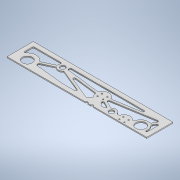
# Autodesk Inventor part: Right left side
Saved by Autodesk Inventor 2021 (Build 250183000, 183)
## iProperties
Created: 2020-09-02
Part Number: Right left side
Material: Generic
Document SubType Name: Modeling
Designer: deli
Density: 1 g/cm^3
Appearance: Default
Author: deli
Autodesk Inventor part; units mm, degrees
ref_plane "YZ Plane" through (0, 0, 0) normal (1, 0, 0) x (0, 1, 0)
ref_plane "XZ Plane" through (0, 0, 0) normal (0, 1, 0) x (-1, 0, 0)
ref_plane "XY Plane" through (0, 0, 0) normal (0, 0, 1) x (1, 0, 0)
sketch "Sketch1" plane through (0, 0, 0) normal (0, 1, 0) x (-1, 0, 0)
  arc A0 (82.9131, -43.5291) -> (113.1279, -37.6957) centre (96.2781, -31.587) ccw
  arc A1 (116.2464, -35.6057) -> (113.1279, -37.6957) centre (116.1128, -38.7779) ccw
  line L0 (116.2464, -35.6057) -> (118.6042, -35.705)
  arc A2 (121.4505, -37.7814) -> (118.6042, -35.705) centre (118.4706, -38.8772) ccw
  arc A3 (121.4505, -37.7814) -> (142.7671, -43.2201) centre (133.978, -33.1745) ccw
  arc A4 (146.2603, -42.7612) -> (142.7671, -43.2201) centre (144.8577, -45.6096) ccw
  line L1 (146.2603, -42.7612) -> (165.8088, -52.3866)
  arc A5 (167.5414, -55.7362) -> (165.8088, -52.3866) centre (164.4062, -55.235) ccw
  arc A6 (167.5414, -55.7362) -> (167.4812, -56.1422) centre (185.6904, -58.637) ccw
  arc A7 (164.8504, -58.8442) -> (167.4812, -56.1422) centre (164.3356, -55.7112) ccw
  line L2 (164.8504, -58.8442) -> (44.4643, -78.6278)
  arc A8 (41.2217, -73.8701) -> (44.4643, -78.6278) centre (43.9495, -75.4948) ccw
  line L3 (41.2217, -73.8701) -> (47.7775, -62.8629)
  arc A9 (51.3513, -61.4274) -> (47.7775, -62.8629) centre (50.5053, -64.4876) ccw
  arc A10 (51.3513, -61.4274) -> (77.4222, -45.0742) centre (56.9081, -41.3279) ccw
  arc A11 (82.9131, -43.5291) -> (77.4222, -45.0742) centre (80.5456, -45.6446) ccw
  line L4 (301.7886, -83.9745) -> (89.9873, -83.9745)
  arc A12 (89.4725, -77.6666) -> (89.9873, -83.9745) centre (89.9873, -80.7995) ccw
  line L5 (89.4725, -77.6666) -> (165.8801, -65.1101)
  arc A13 (169.2372, -66.8281) -> (165.8801, -65.1101) centre (166.395, -68.2431) ccw
  arc A14 (169.2372, -66.8281) -> (202.4809, -66.1121) centre (185.6904, -58.637) ccw
  arc A15 (205.7609, -64.2511) -> (202.4809, -66.1121) centre (205.3815, -67.4034) ccw
  line L6 (205.7609, -64.2511) -> (301.5184, -75.7787)
  arc A16 (304.1949, -78.0698) -> (301.5184, -75.7787) centre (301.139, -78.9309) ccw
  arc A17 (304.1949, -78.0698) -> (304.7197, -79.5793) centre (317.0423, -74.4495) ccw
  arc A18 (301.7886, -83.9745) -> (304.7197, -79.5793) centre (301.7886, -80.7995) ccw
  arc A19 (36.5072, -37.0074) -> (41.8818, -55.7874) centre (56.9081, -41.3279) ccw
  arc A20 (42.3218, -59.6135) -> (41.8818, -55.7874) centre (39.594, -57.9889) ccw
  line L7 (42.3218, -59.6135) -> (37.4109, -67.859)
  arc A21 (31.5081, -66.2343) -> (37.4109, -67.859) centre (34.6831, -66.2343) ccw
  line L8 (31.5081, -66.2343) -> (31.5081, -36.0792)
  arc A22 (33.4011, -33.1745) -> (31.5081, -36.0792) centre (34.6831, -36.0792) ccw
  arc A23 (36.5072, -37.0074) -> (33.4011, -33.1745) centre (33.4011, -36.3495) ccw
  arc A24 (199.2854, -40.8697) -> (205.6208, -34.7422) centre (185.6904, -20.4745) ccw
  arc A25 (209.4092, -33.6537) -> (205.6208, -34.7422) centre (208.2024, -36.5904) ccw
  line L9 (209.4092, -33.6537) -> (272.6057, -59.6223)
  arc A26 (271.0195, -65.7113) -> (272.6057, -59.6223) centre (271.3989, -62.559) ccw
  line L10 (271.0195, -65.7113) -> (206.5199, -57.9466)
  arc A27 (203.7752, -55.3604) -> (206.5199, -57.9466) centre (206.8994, -54.7944) ccw
  arc A28 (203.7752, -55.3604) -> (198.7844, -45.7396) centre (185.6904, -58.637) ccw
  arc A29 (199.2854, -40.8697) -> (198.7844, -45.7396) centre (201.0464, -43.5116) ccw
  line L11 (306.2574, -66.5852) -> (239.8235, -39.2863)
  arc A30 (241.0303, -33.1745) -> (239.8235, -39.2863) centre (241.0303, -36.3495) ccw
  line L12 (241.0303, -33.1745) -> (277.3621, -33.1745)
  arc A31 (277.6891, -33.1914) -> (277.3621, -33.1745) centre (277.3621, -36.3495) ccw
  line L13 (277.6891, -33.1914) -> (359.0687, -41.6169)
  arc A32 (361.8936, -44.392) -> (359.0687, -41.6169) centre (358.7418, -44.775) ccw
  arc A33 (361.8936, -44.392) -> (362.3065, -46.8089) centre (387.1081, -41.3279) ccw
  arc A34 (360.5632, -50.3644) -> (362.3065, -46.8089) centre (359.2063, -47.494) ccw
  line L14 (360.5632, -50.3644) -> (327.4064, -66.0384)
  arc A35 (327.4064, -66.0384) -> (306.2574, -66.5852) centre (317.0423, -74.4495) ccw
  arc A36 (154.7926, -33.1696) -> (153.3885, -39.193) centre (154.791, -36.3446) ccw
  line L15 (154.7926, -33.1696) -> (163.0088, -33.1737)
  arc A37 (165.6085, -34.5282) -> (163.0088, -33.1737) centre (163.0072, -36.3487) ccw
  arc A38 (165.6085, -34.5282) -> (172.0953, -40.8697) centre (185.6904, -20.4745) ccw
  arc A39 (172.5963, -45.7396) -> (172.0953, -40.8697) centre (170.3343, -43.5116) ccw
  arc A40 (172.5963, -45.7396) -> (172.3252, -46.0208) centre (185.6904, -58.637) ccw
  arc A41 (168.6138, -46.6898) -> (172.3252, -46.0208) centre (170.0163, -43.8413) ccw
  line L16 (168.6138, -46.6898) -> (153.3885, -39.193)
  arc A42 (329.3649, -79.5793) -> (330.3752, -73.8209) centre (317.0423, -74.4495) ccw
  arc A43 (332.1898, -70.8009) -> (330.3752, -73.8209) centre (333.5467, -73.6713) ccw
  line L17 (332.1898, -70.8009) -> (363.277, -56.1053)
  arc A44 (367.1311, -57.0148) -> (363.277, -56.1053) centre (364.6339, -58.9757) ccw
  arc A45 (367.1311, -57.0148) -> (406.8636, -57.2928) centre (387.1081, -41.3279) ccw
  arc A46 (412.5081, -59.2885) -> (406.8636, -57.2928) centre (409.3331, -59.2885) ccw
  line L18 (412.5081, -59.2885) -> (412.5081, -80.7995)
  arc A47 (409.3331, -83.9745) -> (412.5081, -80.7995) centre (409.3331, -80.7995) ccw
  line L19 (409.3331, -83.9745) -> (332.2961, -83.9745)
  arc A48 (329.3649, -79.5793) -> (332.2961, -83.9745) centre (332.2961, -80.7995) ccw
  arc A49 (173.8824, -20.4745) -> (181.4983, -20.4745) centre (177.6904, -20.3495) ccw
  line L20 (18.8081, -20.4745) -> (173.8824, -20.4745)
  line L21 (18.8081, -20.4745) -> (18.8081, -96.6745)
  line L22 (18.8081, -96.6745) -> (425.2081, -96.6745)
  line L23 (425.2081, -20.4745) -> (425.2081, -96.6745)
  line L24 (197.4983, -20.4745) -> (425.2081, -20.4745)
  arc A50 (189.8824, -20.4745) -> (197.4983, -20.4745) centre (193.6904, -20.3495) ccw
  line L25 (181.4983, -20.4745) -> (189.8824, -20.4745)
  circle A51 centre (88.6581, -25.5545) radius 1.8542
  circle A52 centre (193.6904, -52.3495) radius 1.8542
  circle A53 centre (193.6904, -64.9245) radius 1.8542
  circle A54 centre (103.8981, -25.5545) radius 1.8542
  circle A55 centre (88.6581, -37.6195) radius 1.8542
  circle A56 centre (177.6904, -52.3495) radius 1.8542
  circle A57 centre (177.6904, -64.9245) radius 1.8542
  circle A58 centre (103.8981, -37.6195) radius 1.8542
  circle A59 centre (317.0423, -74.4495) radius 7.2517
  circle A60 centre (133.978, -33.1745) radius 7.2517
  circle A61 centre (56.9081, -41.3279) radius 14.5034
  circle A62 centre (387.1081, -41.3279) radius 14.5034
  point P0 (0, 0)
  point P1 (18.8081, -50.9113)
  dimension "d2" = 14.5034
  dimension "d3" = 29.0068
  dimension "d4" = 14.5034
  constraints: 102 point on circle, 63 centre point, 52 end point
  measures "d2" diameter of A59
  measures "d3" diameter of A62
  measures "d4" diameter of A60
extrude "Extrusion1" add sketch "Sketch1" along normal blind 3.175
equation "\"d4\" = d2"
body "Solid1"
